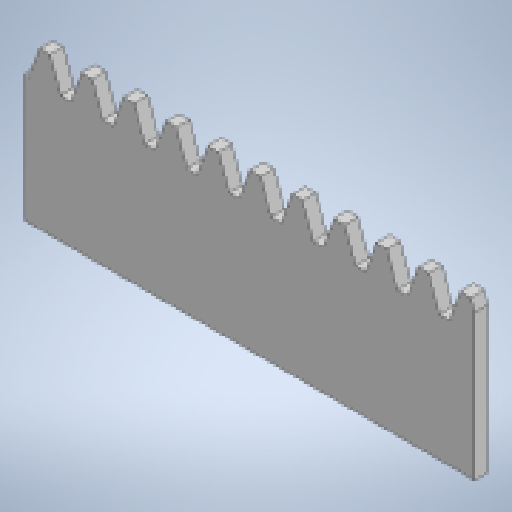
# Autodesk Inventor part: SR3-100_On
Saved by Autodesk Inventor 2024 (Build 280153000, 153)
## iProperties
Created: 2024-06-05
Part Number: SR3-100_On
Material: Generic
Catalog Web Link: www.cadenas.de
Description: Racks (SR)-
Vendor: KHK
Document SubType Name: Modeling
Designer: psAdmin
Manufacturer: KHK
Mass: 95.997 g
Surface Area: 173.548 cm^2
Volume: 95.997 cm^3
Density: 1 g/cm^3
Appearance: PSOLRGB-175-175-175
Category: PARTsolutions
Company: KHK
PSOL_IDENT_0: {$CADENAS_DATA/23d-libs/khk/racks/racks_sr.prj},167 {VTYP=3D},{NB=SR3-100_On},{LINA=SR3-100},{NN=Rac
PSOL_IDENT_1: ks (SR)},{DATE=12.04.2024 02:30:43},{GEOMDATE=26.02.2019 12:12:45},{VERSION=},{LINEID=250},{WBVAR=TO
PSOL_IDENT_2: OTH},{WBNUMERIC=}  {NB=SR3-100_On},{LINA=SR3-100},{KT=DUMMY},{CN=SR3-100},{M=3.0},{A=101},{B=30},{C=
PSOL_IDENT_3: 35.0},{D=32.0},{ENT=9},{S=R1},{WMF=r1004},{TOOTH=On}
NB: SR3-100_On
NN: Racks (SR)
NBSYN: $CN._$TOOTH.
LINA: SR3-100
CATALOG: KHK
CN: SR3-100
M: 3
A: 101
B: 30
C: 35
D: 32
ENT: 9
S: R1
TOOTH: On
SUPPLIER: KHK
ARTICLENO: SR3-100_On
BOMINFO: SR3-100
CREATOR: CADENAS GmbH
Title: SR3-100
Author: Cadenas PARTsolutions
Autodesk Inventor part; units mm, degrees
ref_plane "YZ Plane" through (0, 0, 0) normal (1, 0, 0) x (0, 1, 0)
ref_plane "XZ Plane" through (0, 0, 0) normal (0, 1, 0) x (-1, 0, 0)
ref_plane "XY Plane" through (0, 0, 0) normal (0, 0, 1) x (1, 0, 0)
sketch "Sketch_4" plane through (0, 0, 0) normal (0, 0, 1) x (1, 0, 0)
  line L0 (0, 35) -> (0, 0)
  line L1 (0, 0) -> (101, 0)
  line L2 (101, 0) -> (101, 35)
  line L3 (101, 35) -> (0, 35)
  constraints: 8 end point
extrude "Extrusion1" add sketch "Sketch_4" along normal mid plane 30
sketch "Sketch_5" plane through (0, 0, 0) normal (0, 0, 1) x (1, 0, 0)
  line L0 (-3.5355, 35) -> (-1.1775, 28.25)
  line L1 (-1.1775, 28.25) -> (1.1775, 28.25)
  line L2 (1.1775, 28.25) -> (3.5355, 35)
  line L3 (3.5355, 35) -> (-3.5355, 35)
  constraints: 8 end point
extrude "Extrusion2" cut sketch "Sketch_5" along normal mid plane 30
pattern_linear "Rectangular Pattern1" count 12 spacing 9.4248 along (1, 0, 0) of "Extrusion2"
sketch "スケッチ3" plane through (0, 0, 15) normal (0, -1, 0) x (1, 0, 0)
  line L0 (101, -30) -> (101, 0) projected
  line L1 (0, 0) -> (101, 0) projected
  line L2 (0, -30) -> (0, 0) projected
  line L3 (101, -30) -> (0, -30) projected
  line L4 (0, 0) -> (101, 0) projected
  line L5 (0, 0) -> (101, 0)
  line L6 (101, 0) -> (101, -3)
  line L7 (101, -3) -> (0, -3)
  line L8 (0, -3) -> (0, 0)
  point P0 (0, -15)
  dimension "d10" = 3
  constraints: 8 end point, 2 parallel, 1 horizontal, 1 perpendicular, 1 point on line
  measures "d10" distance of L5.end L6.end
extrude "押し出し3" cut sketch "スケッチ3" against normal through all contours L3 L2 L7 L0
sketch "スケッチ4" plane through (0, 0, 15) normal (0, 0, 1) x (1, 0, 0)
  circle A0 centre (5, 23.25) radius 1.3
  circle A1 centre (5, 23.25) radius 5 construction
  line L0 (0, 28.25) -> (0, 0) projected
  line L1 (1.1775, 28.25) -> (0, 28.25) projected
  line L2 (0, 0) -> (101, 0) projected
  line L3 (50.5, 0) -> (50.5, 28.25) construction
  circle A2 centre (96, 23.25) radius 1.3
  circle A3 centre (96, 23.25) radius 5 construction
  line L4 (99.8225, 28.25) -> (101, 28.25)
  circle A4 centre (50.5, 23.25) radius 1.1
  line L5 (0, 18.25) -> (101, 18.25)
  line L6 (101, 0) -> (101, 32.5295) projected
  dimension "d13" = 2.6
  dimension "d14" = 10
  dimension "d15" = 5
  dimension "d16" = 2.2
  constraints: 6 end point, 5 centre point, 4 symmetric about line, 3 point on line, 2 coincident, 2 tangent, 1 horizontal, 1 horizontal alignment, 1 midpoint, 1 vertical, 2 other
  measures "d13" diameter of A0
  measures "d14" diameter of A1
  measures "d15" distance from line of L1 A1.centre
  measures "d16" diameter of A4
extrude "押し出し4" cut sketch "スケッチ4" against normal through all
body "Solid1"
